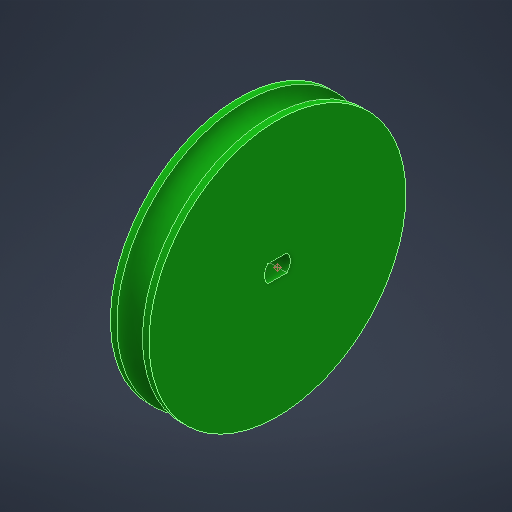
# Autodesk Inventor part: Rodinha-01
Saved by Autodesk Inventor 2026 (Build 300175000, 175)
## iProperties
Created: 2018-07-03
Part Number: Rodinha-01
Material: Genérico
Document SubType Name: Modeling
Designer: Marcelo
Density: 1 g/cm^3
Appearance: Verde escuro
Author: Marcelo
Autodesk Inventor part; units mm, degrees
ref_plane "YZ Plane" through (0, 0, 0) normal (1, 0, 0) x (0, 1, 0)
ref_plane "XZ Plane" through (0, 0, 0) normal (0, 1, 0) x (-1, 0, 0)
sketch "Esboço1" plane through (0, 0, 0) normal (0, 0, 1) x (1, 0, 0)
  line L0 (0, 0) -> (0, 30)
  line L1 (0, 3) -> (-8, 3)
  line L2 (0, 0) -> (2.8421, 0)
  circle A0 centre (-4.5, 30) radius 3
  line L3 (-1.5, 30) -> (0, 30)
  line L4 (-7.5, 30) -> (-9, 30)
  line L5 (-8, 3) -> (-8, 6)
  line L6 (-9, 30) -> (-9, 25)
  line L7 (-9, 25) -> (-8, 25)
  arc A1 (-8, 6) -> (-8, 25) centre (-11.8508, 15.5) ccw
  point P0 (0, 15)
  point P1 (-1.6, 15.5)
  dimension "d1" = 3
  dimension "d3" = 6
  dimension "d4" = 1.5
  dimension "d7" = 1.5
  dimension "d15" = 8
  dimension "d79" = 0
  dimension "d80" = 0
  dimension "d81" = 30
  dimension "d93" = 5
  dimension "d94" = 3
  dimension "d95" = 1.6
  constraints: 16 end point, 5 point on circle, 3 horizontal, 3 vertical, 2 centre point, 2 perpendicular, 2 point on line, 1 midpoint
  measures "d1" distance between parallel lines of L1 L2
  measures "d3" diameter of A0
  measures "d4" distance of L0.end L3.start
  measures "d7" distance of L4.start L4.end
  measures "d15" distance of L1.start L1.end
  measures "d79" distance between parallel lines of L4 L3
  measures "d80" distance from line of L3 A0.centre
  measures "d81" vertical distance of A0.centre L0.start
  measures "d93" distance of L4.end L6.end
  measures "d94" distance of L1.end L5.end
  measures "d95" horizontal distance of point (0, 15) point (-1.6, 15.5)
revolve "Revolução1" add sketch "Esboço1" angle 360 about axis through (0, 0, 0) along (1, 0, 0) contours L1 L5 A1 L7 L6 L4 A0 L3 L0
sketch "Esboço3" plane through (-8, 0, 0) normal (-1, 0, 0) x (0, -1, 0)
  circle A0 centre (0, 0) radius 3 projected
  arc A1 (-2.2361, -2) -> (0, -3) centre (0, 0) ccw
  arc A2 (-2.2361, -2) -> (2.2361, -2) centre (0, 0) ccw
  line L0 (-2.2361, 2) -> (2.2361, 2)
  line L1 (-2.2361, -2) -> (2.2361, -2)
  dimension "d84" = 4
  constraints: 6 point on circle, 4 end point, 2 centre point, 2 coincident, 1 horizontal
  measures "d84" distance between parallel lines of L1 L0
sketch "Esboço6" plane through (-8, 0, 0) normal (-1, 0, 0) x (0, -1, 0)
  circle A0 centre (0, 0) radius 6 projected
  circle A1 centre (0, 0) radius 3
  constraints: 1 centre point, 1 coincident
ref_plane "Plano de trabalho4" through (-4.5, 0, 0) normal (-1, 0, 0) x (0, 0, 1)
extrude "Extrusão9" add sketch "Esboço3" along normal blind 2 and the other way blind 8 contours L0 A0 | A0 L1
extrude "Extrusão10" add sketch "Esboço6" along normal blind 2
fillet "Arredondamento13" radius 2 1 edges at (-10, 6, 0)
equation "\"d23\" = d22"
equation "\"d22\" = 10deg"
